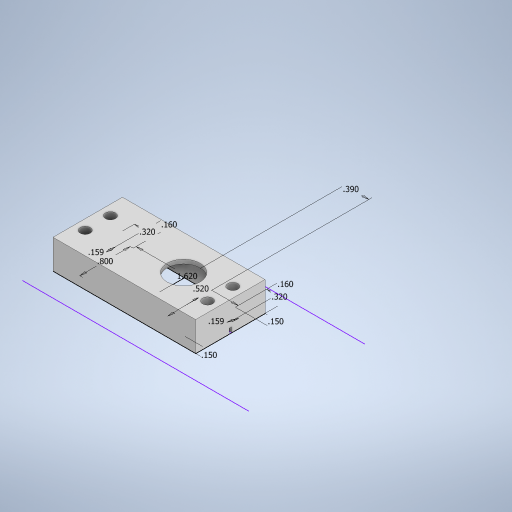
# Autodesk Inventor part: Servo Mount
Saved by Autodesk Inventor 2023 (Build 270158000, 158)
## iProperties
Created: 2023-03-13
Part Number: Servo Mount
Material: Generic
Document SubType Name: Modeling
Designer: tommy
Density: 1 g/cm^3
Appearance: Default
Author: tommy
Autodesk Inventor part; units mm, degrees
ref_plane "YZ Plane" through (0, 0, 0) normal (1, 0, 0) x (0, 1, 0)
ref_plane "XZ Plane" through (0, 0, 0) normal (0, 1, 0) x (-1, 0, 0)
ref_plane "XY Plane" through (0, 0, 0) normal (0, 0, 1) x (1, 0, 0)
sketch "Sketch1" plane through (0, 0, 0) normal (0, 1, 0) x (-1, 0, 0)
  line L0 (0, 0) -> (41.148, 0)
  line L1 (41.148, 0) -> (41.148, -20.32)
  line L2 (41.148, -20.32) -> (0, -20.32)
  line L3 (0, -20.32) -> (0, 0)
  circle A0 centre (45.212, -15.24) radius 2.0193
  circle A1 centre (-4.064, -15.24) radius 2.0193
  circle A2 centre (45.212, -5.08) radius 2.0193
  circle A3 centre (-4.064, -5.08) radius 2.0193
  line L4 (41.148, -9.652) -> (49.276, -9.652)
  line L5 (41.148, -10.668) -> (49.276, -10.668)
  line L6 (-8.128, -9.652) -> (0, -9.652)
  line L7 (-8.128, -10.668) -> (0, -10.668)
  line L8 (-8.128, 3.81) -> (49.276, 3.81)
  line L9 (49.276, 3.81) -> (49.276, -24.13)
  line L10 (49.276, -24.13) -> (-8.128, -24.13)
  line L11 (-8.128, -24.13) -> (-8.128, 3.81)
  line L12 (-6.155, -5.4575) -> (-6.0508, -5.4409)
  line L13 (-6.155, -5.4575) -> (-6.0508, -5.4409)
  line L14 (20.574, -20.32) -> (20.574, 0)
  line L15 (-38.8148, -33.5345) -> (54.3929, -33.5345)
  line L16 (-38.8148, 13.2145) -> (52.2934, 13.2145)
  circle A4 centre (10.668, -10.16) radius 6.604
  point P0 (20.574, -10.16)
  dimension "d0" = 41.148
  dimension "d1" = 20.32
  dimension "d4" = 4.0386
  dimension "d5" = 4.0386
  dimension "d18" = 4.064
  dimension "d19" = 4.064
  dimension "d52" = 8.128
  dimension "d53" = 8.128
  dimension "d54" = 3.81
  dimension "d55" = 3.81
  dimension "d59" = 9.906
  dimension "d60" = 13.208
  constraints: 34 end point, 8 point on line, 4 centre point, 4 horizontal, 4 parallel, 3 midpoint, 2 perpendicular, 1 coincident, 3 other
  measures "d0" distance of L1.end L2.end
  measures "d1" distance of L0.end L1.end
  measures "d4" diameter of A0
  measures "d5" diameter of A1
  measures "d18" distance from line of L1 A0.centre
  measures "d19" distance from line of L3 A1.centre
  measures "d52" distance between parallel lines of L1 L9
  measures "d53" distance between parallel lines of L11 L3
  measures "d54" distance between parallel lines of L2 L10
  measures "d55" distance between parallel lines of L8 L0
  measures "d59" distance of point (20.574, -10.16) point (10.668, -10.16)
  measures "d60" diameter of A4
extrude "Extrusion10" add sketch "Sketch1" along normal blind 11.811
extrude "Extrusion11" cut sketch "Sketch1" along normal blind 10.16 contours L0 L14 L2 L3 | L0 L1 L2 L14
extrude "Extrusion12" cut sketch "Sketch1" along normal blind 2.032 contours L3 L7 L11 L6 | L4 L9 L5 L1
body "Solid4"
